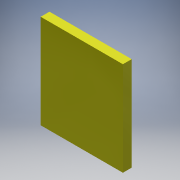
# Autodesk Inventor part: 00_PDMS_mould_0
Saved by Autodesk Inventor 2019.4 (Build 234330000, 330)
## iProperties
Created: 2021-04-19
Part Number: 00_PDMS_mould_0
Material: Generic
Document SubType Name: Modeling
Designer: diederichbenedict
Density: 1 g/cm^3
Appearance: Smooth - Yellow
Author: diederichbenedict
Autodesk Inventor part; units mm, degrees
ref_plane "YZ Plane" through (0, 0, 0) normal (1, 0, 0) x (0, 1, 0)
ref_plane "Work Plane1" through (0, 0, 0) normal (0, 0, 1) x (1, 0, 0)
sketch "Sketch1" plane through (0, 0, 0) normal (0, 0, 1) x (1, 0, 0)
  line L0 (9, 11.7) -> (-9, 11.7) projected
  line L1 (-9, 11.7) -> (-9, -11.7) projected
  line L2 (-9, -11.7) -> (9, -11.7) projected
  line L3 (9, -11.7) -> (9, 11.7) projected
  line L4 (5, -9.05) -> (-2.9937, -9.05) projected
  line L5 (-2.9937, -9.05) -> (-2.9937, -6.1068) projected
  arc A0 (-2.9937, 6.1788) -> (-2.9937, -6.1068) centre (-1.841, 0.036) ccw projected
  line L6 (-2.9937, 6.1788) -> (-2.9937, 9.05) projected
  line L7 (-2.9937, 9.05) -> (5, 9.05) projected
  arc A1 (5, 6.35) -> (5, 9.05) centre (5, 7.7) ccw projected
  line L8 (5, 6.35) -> (0.9246, 6.35) projected
  line L9 (0.9246, 6.35) -> (0.9246, 5.6409) projected
  arc A2 (0.5216, -5.7502) -> (0.9246, 5.6409) centre (-1.841, 0.036) ccw projected
  line L10 (0.5216, -5.7502) -> (0.5216, -6.35) projected
  line L11 (0.5216, -6.35) -> (5, -6.35) projected
  arc A3 (5, -9.05) -> (5, -6.35) centre (5, -7.7) ccw projected
  line L12 (-14, -16) -> (14, -16)
  line L13 (14, -16) -> (14, 16)
  line L14 (14, 16) -> (-14, 16)
  line L15 (-14, 16) -> (-14, -16)
  line L16 (-14, -16) -> (14, 16) construction
  line L17 (14, -16) -> (-14, 16) construction
  point P0 (0, 0)
  dimension "d0" = 28
  dimension "d1" = 32
  constraints: 12 end point, 2 midpoint, 2 parallel, 1 horizontal, 1 perpendicular
  measures "d0" distance of L14.end L13.end
  measures "d1" distance of L13.end L12.end
extrude "Extrusion1" add sketch "Sketch1" along normal blind 3 contours L3 L2 L1 L0 | L4 L5 A0 L6 L7 A1 L8 L9 A2 L10 L11 A3 | L15 L14 L13 L12
sketch "Sketch2" plane through (0, 0, 0) normal (0, 0, -1) x (-1, 0, 0)
  circle A0 centre (1.841, 0.036) radius 6.25 projected
  arc A1 (-5, -9.05) -> (-5, -6.35) centre (-5, -7.7) ccw projected
  line L0 (-0.5216, -6.35) -> (-5, -6.35) projected
  line L1 (-0.5216, -5.7502) -> (-0.5216, -6.35) projected
  arc A2 (-0.5216, -5.7502) -> (2.9937, -6.1068) centre (1.841, 0.036) ccw projected
  line L2 (2.9937, -9.05) -> (2.9937, -6.1068) projected
  line L3 (-5, -9.05) -> (2.9937, -9.05) projected
  arc A3 (2.9937, 6.1788) -> (-0.9246, 5.6409) centre (1.841, 0.036) ccw projected
  line L4 (-0.9246, 6.35) -> (-0.9246, 5.6409) projected
  line L5 (-5, 6.35) -> (-0.9246, 6.35) projected
  arc A4 (-5, 6.35) -> (-5, 9.05) centre (-5, 7.7) ccw projected
  line L6 (2.9937, 9.05) -> (-5, 9.05) projected
  line L7 (2.9937, 6.1788) -> (2.9937, 9.05) projected
  circle A5 centre (-5, 7.7) radius 1.35 projected
  circle A6 centre (-5, -7.7) radius 1.35 projected
  point P0 (0, 0)
ref_plane "Work Plane2" through (-8.091, -6.214, -0.6) normal (0, 0, 1) x (1, 0, 0)
extrude "Extrusion2" add sketch "Sketch2" along normal up to surface (0.6 mm away)
sketch "Sketch3" plane through (5, -9.05, -0.6) normal (0, 0, -1) x (-1, 0, 0)
  circle A0 centre (6.841, 9.086) radius 5 projected
  circle A1 centre (0, 16.75) radius 1.35 projected
  circle A2 centre (0, 1.35) radius 1.35 projected
  point P0 (5, 9.05)
extrude "Extrusion3" add sketch "Sketch3" along normal blind 2
sketch "Sketch4" plane through (-1.841, 0.036, -2.6) normal (0, 0, -1) x (-1, 0, 0)
  circle A0 centre (0, 0) radius 5.2 projected
  point P0 (-1.841, -0.036)
ref_plane "Work Plane3" through (-9, -11.7, -1) normal (0, 0, -1) x (0, 1, 0)
extrude "Extrusion4" cut sketch "Sketch4" against normal up to surface (1.6 mm away)
body "Solid1"
